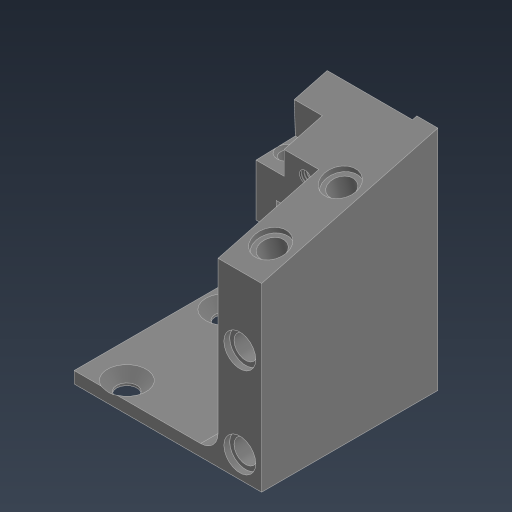
# Autodesk Inventor part: side-right
Saved by Autodesk Inventor 2023 (Build 270158000, 158)
## iProperties
Created: 2025-04-29
Part Number: side-right
Material: Generic
Document SubType Name: Sheet Metal
Designer: szymo
Density: 1 g/cm^3
Appearance: Default(1)
Mass: 8.13192 g
Surface Area: 60.8333 cm^2
Volume: 8.13192 cm^3
Sheet Metal Rule: Default
Author: szymo
Autodesk Inventor part; units mm, degrees
ref_plane "YZ Plane" through (0, 0, 0) normal (1, 0, 0) x (0, 1, 0)
ref_plane "XZ Plane" through (0, 0, 0) normal (0, 1, 0) x (-1, 0, 0)
ref_plane "XY Plane" through (0, 0, 0) normal (0, 0, 1) x (1, 0, 0)
ref_plane "Work Plane1" through (0, 0, 0) normal (0, 0, 1) x (1, 0, 0)
sketch "Sketch1" plane through (0, 0, 0) normal (0, 0, 1) x (1, 0, 0)
  line L0 (-30.025, -43.5645) -> (-17.225, -43.5645) projected
  line L1 (-17.225, -14.8645) -> (-19.375, -14.8645) projected
  arc A0 (-23.375, -10.8645) -> (-19.375, -14.8645) centre (-19.375, -10.8645) ccw projected
  line L2 (-23.375, -10.8645) -> (-23.375, 0.9) projected
  arc A1 (-19.375, 4.9) -> (-23.375, 0.9) centre (-19.375, 0.9) ccw projected
  line L3 (-19.375, 4.9) -> (13.225, 4.9) projected
  arc A2 (17.225, 0.9) -> (13.225, 4.9) centre (13.225, 0.9) ccw projected
  line L4 (17.225, -27.7355) -> (19.375, -27.7355) projected
  arc A3 (23.375, -31.7355) -> (19.375, -27.7355) centre (19.375, -31.7355) ccw projected
  line L5 (23.375, -31.7355) -> (23.375, -43.5645) projected
  line L6 (23.375, -43.5645) -> (30.025, -43.5645) projected
  line L7 (30.025, -43.5645) -> (30.025, 4.9) projected
  line L8 (30.025, 4.9) -> (49.5, 4.9) projected
  line L9 (49.5, 4.9) -> (49.5, 44.0088) projected
  line L10 (45.675, 44.0088) -> (49.5, 44.0088) projected
  line L11 (45.675, 44.0088) -> (45.675, 31.3) projected
  line L12 (45.675, 31.3) -> (35.425, 31.3) projected
  line L13 (35.425, 31.3) -> (35.425, 25.8523) projected
  line L14 (35.425, 25.8523) -> (31, 25.8523) projected
  line L15 (31, 25.8523) -> (31, 31.3) projected
  line L16 (31, 31.3) -> (30.675, 31.3) projected
  line L17 (30.675, 31.3) -> (30.675, 44.0088) projected
  line L18 (4.35, 44.0088) -> (30.675, 44.0088) projected
  line L19 (4.35, 44.0088) -> (4.35, 25.5932) projected
  line L20 (4.35, 25.5932) -> (-4.35, 25.5932) projected
  line L21 (-4.35, 25.5932) -> (-4.35, 44.0088) projected
  line L22 (-30.675, 44.0088) -> (-4.35, 44.0088) projected
  line L23 (-30.675, 44.0088) -> (-30.675, 31.3) projected
  line L24 (-30.675, 31.3) -> (-31, 31.3) projected
  line L25 (-31, 31.3) -> (-31, 25.8523) projected
  line L26 (-31, 25.8523) -> (-35.425, 25.8523) projected
  line L27 (-35.425, 25.8523) -> (-35.425, 31.3) projected
  line L28 (-35.425, 31.3) -> (-45.675, 31.3) projected
  line L29 (-45.675, 31.3) -> (-45.675, 44.0088) projected
  line L30 (-49.5, 44.0088) -> (-45.675, 44.0088) projected
  line L31 (-49.5, 44.0088) -> (-49.5, 4.9) projected
  line L32 (-49.5, 4.9) -> (-30.025, 4.9) projected
  line L33 (-30.025, 4.9) -> (-30.025, -43.5645) projected
  line L34 (17.225, 4.9) -> (28.725, 4.9) projected
  line L35 (28.725, 4.9) -> (30.025, 4.9) projected
  line L36 (17.225, 6.9) -> (46, 6.9)
  line L37 (46, 6.9) -> (46, 44.0088)
  line L38 (46, 44.0088) -> (49.5, 44.0088)
  line L39 (17.225, 6.9) -> (17.225, 4.9)
  circle A4 centre (-45.75, 27.8) radius 1.7 projected
  circle A5 centre (45.75, 8.4) radius 1.7 projected
  circle A6 centre (20.8148, -16.4316) radius 1.7 projected
  circle A7 centre (-22.5007, -33.3594) radius 1.7 projected
  circle A8 centre (-21.409, -21.524) radius 1.7 projected
  circle A9 centre (21.8662, 0.8618) radius 1.7 projected
  circle A10 centre (45.75, 27.8) radius 1.7 projected
  circle A11 centre (-45.75, 8.4) radius 1.7 projected
  line L40 (17.225, -26.7859) -> (17.225, -27.7355) projected
  line L41 (-17.225, -26.7859) -> (-17.225, -43.5645) projected
  line L42 (17.225, -26.7859) -> (-17.225, -26.7859) projected
  line L43 (-17.225, -15.8141) -> (-17.225, -14.8645) projected
  line L44 (17.225, -15.8141) -> (17.225, 0.9) projected
  line L45 (-17.225, -15.8141) -> (17.225, -15.8141) projected
  point P0 (0, 0)
  point P1 (46, 44.0088)
  dimension "d0" = 2
  dimension "d1" = 3.5
  dimension "d2" = 0
  constraints: 9 end point, 4 perpendicular, 1 point on line, 1 other
  measures "d0" distance between parallel lines of L34 L36
  measures "d1" distance between parallel lines of L9 L37
  measures "d2" distance between parallel lines of L10 L38
ref_plane "Work Plane2" through (17.225, -49.9, 30.3429) normal (0, 0, 1) x (1, 0, 0)
extrude "Extrusion1" add sketch "Sketch1" along normal up to surface (30.3429 mm away) contours L35 L34 L39 L36 A5 L37 A10 L10 L9 L8 | A10 L37 | L36 L37 A5 picked at (46.4833, 27.8) picked at (46.1294, 8.9857)
sketch "Sketch2" plane through (49.5, 4.9, 0) normal (1, 0, 0) x (0, 0, -1)
  line L0 (-30.3429, 39.1088) -> (-30.3429, 0) projected
  line L1 (0, 0) -> (-30.3429, 0) projected
  line L2 (0, 0) -> (0, 39.1088) projected
  line L3 (0, 39.1088) -> (-30.3429, 39.1088) projected
  line L4 (-4.1722, 34.5399) -> (-14.667, 34.2101)
  line L5 (0, 39.1088) -> (-30.3429, 31.1137)
  point P0 (0, -4.9)
  point P1 (-9.6486, 34.3678)
  point P2 (-9.1906, 34.3822)
  dimension "d99" = 1
  constraints: 4 end point, 1 point on line, 5 other
  measures "d99" distance from line of L5 L4.end
extrude "Extrusion2" cut sketch "Sketch2" against normal blind 10 contours L3 L5 L0
sketch "Sketch3" plane through (46, 6.9, 0) normal (-1, 0, 0) x (0, 0, 1)
  line L0 (30.3429, 0) -> (23.3429, 0)
  line L1 (30.3429, 29.1137) -> (30.3429, -2) projected
  line L2 (0, 30.9041) -> (30.3429, 22.9089)
  line L3 (23.3429, 24.7534) -> (23.3429, 0)
  line L4 (0, 0) -> (7, 0)
  line L5 (7, 0) -> (7, 5)
  line L6 (7, 5) -> (0, 5)
  line L7 (0, 5) -> (0, 0)
  line L8 (0, 20.5) -> (7, 20.5)
  line L9 (7, 20.5) -> (7, 13.5)
  line L10 (7, 13.5) -> (0, 13.5)
  line L11 (0, 13.5) -> (0, 20.5)
  line L12 (30.3429, 29.1137) -> (0, 37.1088) projected
  line L13 (0, 37.1088) -> (0, 30.9036)
  line L14 (0, 37.1088) -> (0, 0) projected
  point P0 (0, -6.9)
  point P1 (26.8992, 30.0211)
  point P2 (30.3429, 11.6462)
  point P3 (23.3429, 18.6462)
  point P4 (8.2798, 34.9272)
  point P5 (8.2798, 34.9272)
  dimension "d27" = 7
  dimension "d28" = 5
  dimension "d29" = 7
  dimension "d30" = 7
  dimension "d100" = 6
  dimension "d101" = 7
  dimension "d102" = 8.5
  constraints: 24 end point, 8 point on line, 5 parallel, 3 horizontal, 2 perpendicular, 1 coincident, 6 other
  measures "d27" distance of L6.end L5.end
  measures "d28" distance of L5.end L4.end
  measures "d29" distance of L9.end L10.end
  measures "d30" distance of L8.end L9.end
  measures "d100" distance between parallel lines of L12 L2
  measures "d101" distance between parallel lines of L3 L1
  measures "d102" distance between parallel lines of L10 L6
extrude "Extrusion3" add sketch "Sketch3" along normal blind 4
sketch "Sketch4" plane through (46, 6.4, 0) normal (-1, 0, 0) x (0, 0, 1)
  line L0 (0, 5.5) -> (7, 5.5) projected
  line L1 (7, 5.5) -> (7, 0.5) projected
  line L2 (7, 0.5) -> (23.3429, 0.5) projected
  line L3 (23.3429, 0.5) -> (23.3429, 25.2534) projected
  line L4 (23.3429, 25.2534) -> (0, 31.4041) projected
  line L5 (0, 31.4041) -> (0, 21) projected
  line L6 (0, 21) -> (7, 21) projected
  line L7 (7, 21) -> (7, 14) projected
  line L8 (7, 14) -> (0, 14) projected
  line L9 (0, 14) -> (0, 5.5) projected
  line L10 (30.3429, 29.6137) -> (0, 37.6088) projected
  line L11 (0, 37.6088) -> (0, 31.4041) projected
  line L12 (0, 31.4041) -> (23.3429, 25.2534) projected
  line L13 (23.3429, 25.2534) -> (23.3429, 0.5) projected
  line L14 (30.3429, 0.5) -> (23.3429, 0.5) projected
  line L15 (30.3429, 0.5) -> (30.3429, 29.6137) projected
  line L16 (0.75, 24.9) -> (3.5, 24.9)
  line L17 (0.75, 32.65) -> (0.75, 30.15)
  line L18 (0, 37.6088) -> (30.3429, 29.6137) projected
  line L19 (13, 34.1834) -> (13, 25.9)
  line L20 (13, 25.9) -> (0, 25.9)
  line L21 (0, -1.5) -> (0, 37.6088) projected
  line L22 (0.75, 24.9) -> (4.7854, 24.9)
  point P0 (0, 25.9)
  point P1 (13, 34.1834)
  dimension "d103" = 1
  dimension "d104" = 13
  constraints: 10 end point, 2 horizontal, 2 point on line, 2 vertical, 5 other
  measures "d103" distance between parallel lines of L20 L22
  measures "d104" distance between parallel lines of L11 L19
extrude "Extrusion4" add sketch "Sketch4" along normal blind 14.8 contours L5 L4 L19 L20 | L11 L10 L19 L4
sketch "Sketch13" plane through (31.2, 6.4, 0) normal (-1, 0, 0) x (0, 0, 1)
  line L0 (0.75, 21.9) -> (0.75, 35.9)
  line L1 (0, 25.9) -> (13, 25.9) projected
  line L2 (13, 25.9) -> (13, 34.1834) projected
  line L3 (13, 34.1834) -> (0, 37.6088) projected
  line L4 (0, 37.6088) -> (0, 25.9) projected
  line L5 (0.75, 35.9) -> (0.75, 37.4112)
  line L6 (0.75, 21.9) -> (0.75, 21)
  line L7 (0.75, 21) -> (0, 21)
  line L8 (0, 21) -> (0, 25.9)
  line L9 (7, 21) -> (0, 21) projected
  point P0 (0, -6.4)
  point P1 (0.75, 25.9)
  constraints: 10 end point, 2 perpendicular, 2 point on line, 2 vertical, 1 collinear, 2 other
extrude "Extrusion8" cut sketch "Sketch13" against normal blind 14.675 contours L6 L7 L8 L1 L0 | L1 L4 L3 L5 L0
sketch "Sketch14" plane through (31.2, 6.4, 0) normal (-1, 0, 0) x (0, 0, 1)
  line L0 (0.75, 37.4112) -> (0.75, 25.9) projected
  line L1 (0.75, 25.9) -> (13, 25.9) projected
  line L2 (13, 25.9) -> (13, 34.1834) projected
  line L3 (13, 34.1834) -> (0.75, 37.4112) projected
  line L4 (10.095, 19.3471) -> (7.8961, 19.4162)
  line L5 (10.1578, 21.3461) -> (7.9589, 21.4152)
  line L6 (7.9589, 21.4152) -> (7.8961, 19.4162)
  line L7 (10.1578, 21.3461) -> (10.095, 19.3471)
  line L8 (6.2339, 21.4694) -> (6.2339, 25.9)
  line L9 (13, 25.9) -> (0.75, 25.9) projected
  line L10 (6.2339, 21.4694) -> (13, 21.2568)
  line L11 (6.2339, 21.4694) -> (1.8033, 25.9)
  line L12 (13, 21.2568) -> (13, 25.9)
  point P0 (0, -6.4)
  dimension "d108" = 45
  dimension "d109" = 1.725
  constraints: 16 end point, 3 perpendicular, 3 point on line, 1 collinear, 6 other
  measures "d108" angle of L1 L11
  measures "d109" horizontal distance of L8.start L5.end
extrude "Extrusion9" add sketch "Sketch14" against normal blind 3.45 contours L12 L10 L5 L8 L1
sketch "Sketch10" plane through (0, 0, 0) normal (0, 0, -1) x (-1, 0, 0)
  line L0 (-45.675, 44.0088) -> (-45.675, 31.3) projected
  line L1 (-30.675, 31.3) -> (-30.675, 44.0088) projected
  line L2 (-45.675, 44.0088) -> (-30.675, 44.0088)
  line L3 (-49.5, 44.0088) -> (-46, 44.0088) projected
  line L4 (-30.675, 31.3) -> (-45.675, 31.3)
  line L5 (-46, 27.4) -> (-42, 27.4) projected
  line L6 (-46, 44.0088) -> (-46, 6.9) projected
  line L7 (-46, 38.5917) -> (-42, 38.5917) projected
  line L8 (-46, 38.5917) -> (-46, 44.0088)
  point P0 (0, 0)
  point P1 (-42, 44.0088)
  point P2 (-45.675, 38.5917)
  constraints: 5 end point, 1 collinear, 1 perpendicular, 4 other
ref_plane "Work Plane4" through (17.675, 44.0069, 10.0686) normal (0, -0.9995066, -0.0314108) x (1, 0, 0)
sketch "Sketch15" plane through (17.675, 44.0069, 10.0686) normal (0, -0.9995066, -0.0314108) x (1, 0, 0)
  circle A0 centre (15.25, -0.5) radius 1.1
  line L0 (28.2, -10.0637) -> (28.2, -9.3078) projected
  line L1 (28.2, -9.3078) -> (13.525, -9.3078) projected
  line L2 (13.525, 3.0375) -> (13.525, -9.3078) projected
  line L3 (24.325, 3.0375) -> (13.525, 3.0375) projected
  line L4 (24.325, 20.5154) -> (24.325, 3.0375) projected
  line L5 (31.825, 20.5154) -> (24.325, 20.5154) projected
  line L6 (31.825, -10.0637) -> (31.825, 20.5154) projected
  line L7 (31.825, -10.0637) -> (28.2, -10.0637) projected
  line L8 (18.35, 3.0375) -> (18.35, -3.6)
  line L9 (18.35, -3.6) -> (13.525, -3.6)
  line L10 (18.35, 3.0375) -> (13.525, 3.0375)
  line L11 (13.525, 3.0375) -> (13.525, 4.5316)
  line L12 (13.525, 4.5316) -> (18.35, 4.5316)
  line L13 (18.35, 4.5316) -> (18.35, 3.0375)
  point P0 (-17.675, -8.6813)
  dimension "d112" = 2
  dimension "d113" = 2
  dimension "d114" = 4.825
  dimension "d115" = 6.6375
  constraints: 12 end point, 4 parallel, 3 point on line, 1 centre point, 1 horizontal, 1 perpendicular, 2 other
  measures "d112" distance edge to line of A0 L9
  measures "d113" distance edge to line of A0 L8
  measures "d114" distance between parallel lines of L8 L2
  measures "d115" distance between parallel lines of L3 L9
extrude "Extrusion10" cut sketch "Sketch15" along normal blind 7.323 contours A0 | L2 L3 L8 L9 | L11 L12 L13 L3
sketch "Sketch16" plane through (17.675, 36.6875, 9.8385) normal (0, 0.9995066, 0.0314108) x (1, 0, 0)
  circle A0 centre (15.25, 0.5) radius 1.1
  point P0 (-17.675, 8.6813)
  constraints: 1 centre point, 1 coincident, 2 other
hole "Hole6" at (32.925, 36.7032, 9.3388) direction (0, -0.9995066, -0.0314108) diameter 2.5 depth 12.048 clearance for "Countersunk Flat Head Screw ISO 2009/7046" size "M2.5" standard "ISO"
chamfer "Chamfer4" distance 0.5 angle 45 1 edges at (32.925, 36.7405, 8.0893)
sketch "Sketch6" plane through (0, 0, 0) normal (0, 0, -1) x (-1, 0, 0)
  circle A0 centre (-39.675, 38.3) radius 1.25
  constraints: 1 centre point, 1 coincident, 2 other
hole "Hole2" at (39.675, 38.3, 0) direction (0, 0, 1) diameter 2.013 depth 17.6 thread size "M2.5x0.45" class "6H" standard "ISO Metric profile"
chamfer "Chamfer5" distance 1 angle 45 1 edges at (39.675, 37.2935, 0.75)
ref_plane "Work Plane3" through (31.175, 31.8, 0.75) normal (0, 0, 1) x (1, 0, 0)
sketch "Sketch5" plane through (0, 0, 0) normal (0, 0, -1) x (-1, 0, 0)
  line L0 (-17.225, 6.9) -> (-17.225, 4.9) projected
  line L1 (-42, 6.9) -> (-17.225, 6.9) projected
  line L2 (-17.225, 4.9) -> (-49.5, 4.9) projected
  line L3 (-46, 27.4) -> (-42, 27.4) projected
  line L4 (-49.5, 36.0137) -> (-49.5, 4.9) projected
  line L5 (-42, 27.4) -> (-49.5, 27.4)
  line L6 (-49.5, 27.4) -> (-49.5, 20.4)
  line L7 (-49.5, 20.4) -> (-42, 20.4)
  line L8 (-42, 20.4) -> (-42, 27.4)
  line L9 (-42, 11.9) -> (-49.5, 11.9)
  line L10 (-49.5, 11.9) -> (-49.5, 4.9)
  line L11 (-49.5, 4.9) -> (-42, 4.9)
  line L12 (-42, 4.9) -> (-42, 11.9)
  line L13 (-42, 27.4) -> (-49.5, 20.4)
  line L14 (-17.225, 4.9) -> (-49.5, 4.9)
  line L15 (-42, 4.9) -> (-49.5, 11.9)
  line L16 (-42, 20.4) -> (-49.5, 27.4)
  line L17 (-49.5, 4.9) -> (-17.225, 4.9)
  line L18 (-46, 20.4) -> (-46, 11.9) projected
  line L19 (-49.5, 44.0088) -> (-45.875, 44.0088) projected
  line L20 (-49.5, 4.9) -> (-49.5, 44.0088) projected
  line L21 (-42, 11.9) -> (-42, 6.9) projected
  line L22 (-46, 11.9) -> (-42, 11.9) projected
  line L23 (-46, 20.4) -> (-42, 20.4) projected
  line L24 (-42, 27.4) -> (-42, 20.4) projected
  line L25 (-45.875, 32.3) -> (-45.875, 44.0088) projected
  line L26 (-46, 27.4) -> (-42, 27.4) projected
  line L27 (-46, 32.3) -> (-46, 27.4) projected
  line L28 (-46, 32.3) -> (-45.875, 32.3) projected
  point P0 (0, 0)
  point P1 (-49.5, 32.1662)
  point P2 (-45.75, 20.4)
  point P3 (-45.75, 23.9)
  point P4 (-45.75, 8.4)
  constraints: 26 end point, 4 parallel, 3 midpoint, 2 horizontal, 2 perpendicular, 1 point on line
hole "Hole1" at (45.75, 23.9, 0) at (45.75, 8.4, 0) direction (0, 0, 1) diameter 4 depth 6 counterbore diameter 5.5 counterbore depth 1
sketch "Sketch7" plane through (42, 35.7639, 31.2909) normal (0, 0.9669949, 0.2547957) x (1, 0, 0)
  line L0 (-5.975, 25.7263) -> (-5.975, 18.9152) projected
  line L1 (0, 18.9152) -> (-5.975, 18.9152) projected
  line L2 (0, 0.9803) -> (0, 18.9152) projected
  line L3 (7.5, 0.9803) -> (0, 0.9803) projected
  line L4 (7.5, 32.3589) -> (7.5, 0.9803) projected
  line L5 (7.5, 32.3589) -> (3.875, 32.3589) projected
  line L6 (3.875, 32.3589) -> (3.875, 31.5833) projected
  line L7 (3.875, 31.5833) -> (-10.8, 31.5833) projected
  line L8 (-10.8, 25.7263) -> (-10.8, 31.5833) projected
  line L9 (-10.8, 25.7263) -> (-5.975, 25.7263) projected
  line L10 (7.5, 22.3589) -> (0, 22.3589)
  line L11 (0, 26.3435) -> (0, 19.5745) projected
  line L12 (0, 18.9152) -> (0, 22.3589)
  circle A0 centre (3.75, 18.8589) radius 3.5
  circle A1 centre (3.75, 6.4803) radius 3.5
  point P0 (-42, 21.1456)
  dimension "d131" = 10
  dimension "d132" = 3.75
  dimension "d133" = 3.75
  dimension "d134" = 3.75
  dimension "d135" = 3.75
  dimension "d136" = 7
  dimension "d137" = 7
  dimension "d138" = 2
  dimension "d139" = 0
  dimension "d140" = 5.3786
  constraints: 4 end point, 2 centre point, 2 coincident, 2 point on line, 1 horizontal, 1 perpendicular
  measures "d131" distance between parallel lines of L5 L10
  measures "d132" distance from line of L4 point (3.75, 6.48)
  measures "d133" distance from line of point (3.75, 6.48) L2
  measures "d134" distance from line of L4 point (3.75, 18.859)
  measures "d135" distance from line of point (3.75, 18.859) L2
  measures "d136" diameter of A0
  measures "d137" diameter of A1
  measures "d138" distance edge to line of A1 L3
  measures "d139" distance edge to line of A0 L10
hole "Hole3" at (45.75, 40.5691, 13.0544) at (45.75, 37.4151, 25.0245) direction (0, -0.9669949, -0.2547957) diameter 4 depth 5 counterbore diameter 5.5 counterbore depth 1
sketch "Sketch8" plane through (17.225, 4.9, 30.3429) normal (0, 0, 1) x (1, 0, 0)
  line L0 (0, 2) -> (24.775, 2) projected
  line L1 (0, 0) -> (0, 2) projected
  line L2 (32.275, 0) -> (0, 0) projected
  circle A0 centre (28.525, 3.75) radius 3.75
  circle A1 centre (28.525, 19.2662) radius 3.5
  line L3 (32.275, 31.1137) -> (24.775, 31.1137) projected
  line L4 (32.275, 31.1137) -> (32.275, 0) projected
  line L5 (24.775, 2) -> (24.775, 31.1137) projected
  point P0 (-17.225, -4.9)
  dimension "d60" = 7.5
  dimension "d61" = 7
  dimension "d62" = 3.75
  constraints: 2 centre point
  measures "d60" diameter of A0
  measures "d61" diameter of A1
  measures "d62" distance from line of L2 A0.centre
hole "Hole4" at (45.75, 8.65, 30.3429) at (45.75, 24.1662, 30.3429) direction (0, 0, -1) diameter 4 depth 5 counterbore diameter 5.5 counterbore depth 1
sketch "Sketch9" plane through (17.225, 6.9, 30.3429) normal (0, 1, 0) x (1, 0, 0)
  circle A0 centre (6.0165, 3.054) radius 2.75 projected
  circle A1 centre (3.9111, 22.1116) radius 2.75 projected
  line L0 (0, 0) -> (0, 30.3429) projected
  line L1 (0, 0) -> (11.5, 0) projected
  line L2 (11.5, 30.3429) -> (11.5, 0) projected
  line L3 (0, 30.3429) -> (11.5, 30.3429) projected
  point P0 (-17.225, 30.3429)
hole "Hole5" at (23.2415, 6.9, 27.289) at (21.1361, 6.9, 8.2313) direction (0, -1, 0) diameter 3.5 depth 5 countersink diameter 6.7 countersink angle 90
fillet "Fillet2" radius 3 11 edges at (46, 6.9, 15.1715) (42, 6.9, 3.5) (42, 6.9, 26.8429) (46, 11.9, 3.5) (42, 11.9, 3.5) (42, 27.4, 3.5) (46, 20.4, 3.5) (42, 20.4, 3.5) (46, 33.016, 18.1715) (32.925, 32.3, 6.2339) (46, 32.3, 6.5)
fillet "Fillet3" radius 1 1 edges at (46, 27.4, 3.5)
equation "\"d62\" = 0.5 * d60"
body "Solid1"
